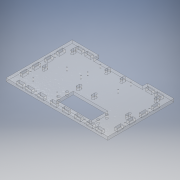
# Autodesk Inventor part: case_base
Saved by Autodesk Inventor 2019 (Build 230136000, 136)
## iProperties
Created: 2019-02-02
Part Number: case_base
Material: Acrylic, Clear
Document SubType Name: Modeling
Designer: suchanek
Density: 1.19 g/cm^3
Appearance: Transparent - Clear
Author: suchanek
Autodesk Inventor part; units mm, degrees
ref_plane "YZ Plane" through (0, 0, 0) normal (1, 0, 0) x (0, 1, 0)
ref_plane "XZ Plane" through (0, 0, 0) normal (0, 1, 0) x (-1, 0, 0)
ref_plane "XY Plane" through (0, 0, 0) normal (0, 0, 1) x (1, 0, 0)
sketch "Sketch1" plane through (0, 0, 0) normal (0, 1, 0) x (-1, 0, 0)
  line L0 (100, 65) -> (-100, 65)
  line L1 (-100, 65) -> (-100, -65)
  line L2 (-100, -65) -> (100, -65)
  line L3 (100, -65) -> (100, 65)
  line L4 (100, 65) -> (-100, -65) construction
  line L5 (-100, 65) -> (100, -65) construction
  line L6 (0, 0) -> (4.5236, 0)
  line L7 (0, 8.9) -> (0, -17.1)
  circle A0 centre (58.5, -13.1) radius 0.9
  circle A1 centre (30.6, -13.1) radius 0.9
  circle A2 centre (73.7, 37.7) radius 0.9
  circle A3 centre (25.5, 39) radius 0.9
  circle A4 centre (15, 6.45) radius 2.4
  line L8 (0, 0) -> (5.2635, 0)
  circle A5 centre (-15, 6.45) radius 2.4
  line L9 (48.5, 0) -> (48.5, 8.2763)
  line L10 (-48.5, 0) -> (-48.5, 8.2763)
  circle A6 centre (-82, 6.45) radius 2.4
  circle A7 centre (82, 6.45) radius 2.4
  line L11 (95.55, -41.85) -> (90.45, -41.85)
  line L12 (90.45, -41.85) -> (90.45, -30.15)
  line L13 (90.45, -30.15) -> (95.55, -30.15)
  line L14 (95.55, -30.15) -> (95.55, -41.85)
  line L15 (95.55, -17.85) -> (90.45, -17.85)
  line L16 (90.45, -17.85) -> (90.45, -6.15)
  line L17 (90.45, -6.15) -> (95.55, -6.15)
  line L18 (95.55, -6.15) -> (95.55, -17.85)
  line L19 (65.85, -55.45) -> (54.15, -55.45)
  line L20 (54.15, -55.45) -> (54.15, -60.55)
  line L21 (54.15, -60.55) -> (65.85, -60.55)
  line L22 (65.85, -60.55) -> (65.85, -55.45)
  line L23 (72.15, -60.55) -> (83.85, -60.55)
  line L24 (83.85, -60.55) -> (83.85, -55.45)
  line L25 (83.85, -55.45) -> (72.15, -55.45)
  line L26 (72.15, -55.45) -> (72.15, -60.55)
  line L27 (-95.55, -41.85) -> (-90.45, -41.85)
  line L28 (-90.45, -41.85) -> (-90.45, -30.15)
  line L29 (-90.45, -30.15) -> (-95.55, -30.15)
  line L30 (-95.55, -30.15) -> (-95.55, -41.85)
  line L31 (-95.55, -17.85) -> (-90.45, -17.85)
  line L32 (-90.45, -17.85) -> (-90.45, -6.15)
  line L33 (-90.45, -6.15) -> (-95.55, -6.15)
  line L34 (-95.55, -6.15) -> (-95.55, -17.85)
  line L35 (-65.85, -55.45) -> (-54.15, -55.45)
  line L36 (-54.15, -55.45) -> (-54.15, -60.55)
  line L37 (-54.15, -60.55) -> (-65.85, -60.55)
  line L38 (-65.85, -60.55) -> (-65.85, -55.45)
  line L39 (-72.15, -60.55) -> (-83.85, -60.55)
  line L40 (-83.85, -60.55) -> (-83.85, -55.45)
  line L41 (-83.85, -55.45) -> (-72.15, -55.45)
  line L42 (-72.15, -55.45) -> (-72.15, -60.55)
  line L43 (95.55, 41.85) -> (90.45, 41.85)
  line L44 (90.45, 41.85) -> (90.45, 30.15)
  line L45 (90.45, 30.15) -> (95.55, 30.15)
  line L46 (95.55, 30.15) -> (95.55, 41.85)
  line L47 (95.55, 17.85) -> (90.45, 17.85)
  line L48 (90.45, 17.85) -> (90.45, 6.15)
  line L49 (90.45, 6.15) -> (95.55, 6.15)
  line L50 (95.55, 6.15) -> (95.55, 17.85)
  line L51 (65.85, 55.45) -> (54.15, 55.45)
  line L52 (54.15, 55.45) -> (54.15, 60.55)
  line L53 (54.15, 60.55) -> (65.85, 60.55)
  line L54 (65.85, 60.55) -> (65.85, 55.45)
  line L55 (41.85, 55.45) -> (30.15, 55.45)
  line L56 (30.15, 55.45) -> (30.15, 60.55)
  line L57 (30.15, 60.55) -> (41.85, 60.55)
  line L58 (41.85, 60.55) -> (41.85, 55.45)
  line L59 (17.85, 55.45) -> (6.15, 55.45)
  line L60 (6.15, 55.45) -> (6.15, 60.55)
  line L61 (6.15, 60.55) -> (17.85, 60.55)
  line L62 (17.85, 60.55) -> (17.85, 55.45)
  line L63 (72.15, 60.55) -> (83.85, 60.55)
  line L64 (83.85, 60.55) -> (83.85, 55.45)
  line L65 (83.85, 55.45) -> (72.15, 55.45)
  line L66 (72.15, 55.45) -> (72.15, 60.55)
  line L67 (-90.45, 30.15) -> (-95.55, 30.15)
  line L68 (-95.55, 17.85) -> (-90.45, 17.85)
  line L69 (-90.45, 17.85) -> (-90.45, 6.15)
  line L70 (-90.45, 6.15) -> (-95.55, 6.15)
  line L71 (-95.55, 6.15) -> (-95.55, 17.85)
  line L72 (-95.55, 41.85) -> (-90.45, 41.85)
  line L73 (-95.55, 30.15) -> (-95.55, 41.85)
  line L74 (-90.45, 41.85) -> (-90.45, 30.15)
  line L75 (-83.85, 55.45) -> (-72.15, 55.45)
  line L76 (-83.85, 60.55) -> (-83.85, 55.45)
  line L77 (-72.15, 60.55) -> (-83.85, 60.55)
  line L78 (-72.15, 55.45) -> (-72.15, 60.55)
  line L79 (-65.85, 60.55) -> (-65.85, 55.45)
  line L80 (-54.15, 55.45) -> (-54.15, 60.55)
  line L81 (-54.15, 60.55) -> (-65.85, 60.55)
  line L82 (-65.85, 55.45) -> (-54.15, 55.45)
  line L83 (-6.15, 55.45) -> (-6.15, 60.55)
  line L84 (-17.85, 55.45) -> (-6.15, 55.45)
  line L85 (-6.15, 60.55) -> (-17.85, 60.55)
  line L86 (-17.85, 60.55) -> (-17.85, 55.45)
  line L87 (-30.15, 55.45) -> (-30.15, 60.55)
  line L88 (-41.85, 60.55) -> (-41.85, 55.45)
  line L89 (-30.15, 60.55) -> (-41.85, 60.55)
  line L90 (-41.85, 55.45) -> (-30.15, 55.45)
  line L91 (82, 3.95) -> (82, 8.95) construction
  line L92 (84.4, 3.95) -> (84.4, 8.95)
  line L93 (79.6, 8.95) -> (79.6, 3.95)
  arc A8 (79.6, 3.95) -> (84.4, 3.95) centre (82, 3.95) ccw
  arc A9 (84.4, 8.95) -> (79.6, 8.95) centre (82, 8.95) ccw
  line L94 (12.6, 3.95) -> (12.6, 8.95)
  line L95 (17.4, 8.95) -> (17.4, 3.95)
  arc A10 (12.6, 3.95) -> (17.4, 3.95) centre (15, 3.95) ccw
  arc A11 (17.4, 8.95) -> (12.6, 8.95) centre (15, 8.95) ccw
  line L96 (-84.4, 3.95) -> (-84.4, 8.95)
  line L97 (-79.6, 8.95) -> (-79.6, 3.95)
  arc A12 (-84.4, 3.95) -> (-79.6, 3.95) centre (-82, 3.95) ccw
  arc A13 (-79.6, 8.95) -> (-84.4, 8.95) centre (-82, 8.95) ccw
  arc A14 (-17.4, 3.95) -> (-12.6, 3.95) centre (-15, 3.95) ccw
  line L98 (-12.6, 3.95) -> (-12.6, 8.95)
  line L99 (-17.4, 8.95) -> (-17.4, 3.95)
  arc A15 (-12.6, 8.95) -> (-17.4, 8.95) centre (-15, 8.95) ccw
  line L100 (-56.5, 53.45) -> (11.5, 53.45)
  line L101 (11.5, 53.45) -> (11.5, 21.45)
  line L102 (11.5, 21.45) -> (-56.5, 21.45)
  line L103 (-56.5, 21.45) -> (-56.5, 53.45)
  circle A16 centre (-61.5, 28.45) radius 2.5
  circle A17 centre (-61.5, 45.45) radius 2.5
  line L104 (47.85, -65) -> (-47.85, -65)
  line L105 (-47.85, -65) -> (-47.85, -55.45)
  line L106 (-47.85, -55.45) -> (47.85, -55.45)
  line L107 (47.85, -55.45) -> (47.85, -65)
  line L108 (-22.5, 6.9) -> (-22.5, -4.1)
  circle A18 centre (16.5, 28.45) radius 2.5
  circle A19 centre (16.5, 45.45) radius 2.5
  circle A20 centre (30, -50.45) radius 0.9
  circle A21 centre (30, -25.45) radius 0.9
  circle A22 centre (-30, -25.45) radius 0.9
  circle A23 centre (-30, -50.45) radius 0.9
  circle A24 centre (93, -24) radius 1.125
  circle A25 centre (93, 24) radius 1.125
  circle A26 centre (-93, -24) radius 1.125
  circle A27 centre (-93, 24) radius 1.125
  circle A28 centre (48, 58) radius 1.125
  circle A29 centre (-48, 58) radius 1.125
  line L109 (65.3403, -21.55) -> (57.8403, -21.55)
  circle A30 centre (15, -49.55) radius 2.4
  circle A31 centre (-15, -49.55) radius 2.4
  circle A32 centre (-82, -49.55) radius 2.4
  circle A33 centre (82, -49.55) radius 2.4
  line L110 (82, -47.05) -> (82, -52.05) construction
  line L111 (84.4, -47.05) -> (84.4, -52.05)
  line L112 (79.6, -52.05) -> (79.6, -47.05)
  arc A34 (84.4, -47.05) -> (79.6, -47.05) centre (82, -47.05) ccw
  arc A35 (79.6, -52.05) -> (84.4, -52.05) centre (82, -52.05) ccw
  arc A36 (17.4, -47.05) -> (12.6, -47.05) centre (15, -47.05) ccw
  line L113 (12.6, -47.05) -> (12.6, -52.05)
  line L114 (17.4, -52.05) -> (17.4, -47.05)
  arc A37 (12.6, -52.05) -> (17.4, -52.05) centre (15, -52.05) ccw
  line L115 (-84.4, -47.05) -> (-84.4, -52.05)
  arc A38 (-84.4, -52.05) -> (-79.6, -52.05) centre (-82, -52.05) ccw
  line L116 (-79.6, -52.05) -> (-79.6, -47.05)
  arc A39 (-79.6, -47.05) -> (-84.4, -47.05) centre (-82, -47.05) ccw
  arc A40 (-12.6, -47.05) -> (-17.4, -47.05) centre (-15, -47.05) ccw
  line L117 (-17.4, -52.05) -> (-17.4, -47.05)
  line L118 (-12.6, -47.05) -> (-12.6, -52.05)
  arc A41 (-17.4, -52.05) -> (-12.6, -52.05) centre (-15, -52.05) ccw
  point P0 (0, 0)
  point P1 (0, 0)
  dimension "d0" = 130
  dimension "d1" = 200
  dimension "d7" = 1.8
  dimension "d8" = 5.1
  dimension "d9" = 27.9
  dimension "d10" = 1.3
  dimension "d11" = 50.8
  dimension "d12" = 15.2
  dimension "d14" = 26
  dimension "d23" = 4.8
  dimension "d31" = 5.1
  dimension "d32" = 4.45
  dimension "d34" = 6.15
  dimension "d35" = 11.7
  dimension "d36" = 12.3
  dimension "d37" = 11.7
  dimension "d43" = 11.7
  dimension "d44" = 6.3
  dimension "d45" = 11.7
  dimension "d50" = 2.5
  dimension "d54" = 10.5
  dimension "d55" = 32
  dimension "d56" = 68
  dimension "d58" = 5
  dimension "d62" = 17
  dimension "d63" = 5
  dimension "d64" = 12.3
  dimension "d65" = 11.7
  dimension "d66" = 5.1
  dimension "d67" = 12.3
  dimension "d68" = 11.7
  dimension "d69" = 12.3
  dimension "d70" = 11.7
  dimension "d71" = 12.3
  dimension "d72" = 11.7
  dimension "d73" = 4.45
  dimension "d74" = 6.3
  dimension "d75" = 6.3
  dimension "d77" = 15
  dimension "d78" = 67
  dimension "d79" = 5
  dimension "d80" = 25
  dimension "d81" = 60
  dimension "d82" = 2.25
  dimension "d83" = 6.15
  dimension "d84" = 2.55
  dimension "d85" = 2.25
  dimension "d86" = 2.25
  dimension "d87" = 2.55
  dimension "d88" = 6.15
  dimension "d89" = 7
  dimension "d90" = 56
  dimension "d91" = 15
  dimension "d92" = 2
  dimension "d93" = 22.5
  constraints: 242 end point, 104 symmetric about line, 42 centre point, 32 point on circle, 16 parallel, 14 point on line, 10 collinear, 10 horizontal, 8 equal radius, 8 vertical, 7 midpoint, 7 perpendicular, 5 tangent, 4 horizontal alignment, 3 vertical alignment, 28 other
  measures "d0" distance of L2.end L0.start
  measures "d1" distance of L1.end L2.end
  measures "d7" diameter of A1
  measures "d8" horizontal distance of A3.centre A1.centre
  measures "d9" distance of A1.centre A0.centre
  measures "d10" vertical distance of A2.centre A3.centre
  measures "d11" vertical distance of A0.centre A2.centre
  measures "d12" horizontal distance of A2.centre A0.centre
  measures "d14" distance from line of L0 A3.centre
  measures "d23" diameter of A4
  measures "d31" distance between parallel lines of L16 L18
  measures "d32" distance between parallel lines of L3 L18
  measures "d34" distance between parallel lines of L17 L8
  measures "d35" distance of L17.end L15.start
  measures "d36" distance between parallel lines of L15 L13
  measures "d37" distance of L13.end L11.start
  measures "d43" distance of L19.start L19.end
  measures "d44" distance between parallel lines of L22 L26
  measures "d45" distance of L24.end L25.end
  measures "d50" distance of A7.centre L91.end
  measures "d54" horizontal distance of A4.centre A3.centre
  measures "d55" distance of L100.end L101.end
  measures "d56" distance of L101.end L102.end
  measures "d58" distance from line of L103 A17.centre
  measures "d62" distance of A16.centre A17.centre
  measures "d63" diameter of A17
  measures "d64" distance between parallel lines of L58 L52
  measures "d65" distance of L56.end L58.start
  measures "d66" distance of L56.start L56.end
  measures "d67" distance between parallel lines of L62 L56
  measures "d68" distance of L61.start L62.start
  measures "d69" distance between parallel lines of L83 L60
  measures "d70" distance of L83.end L85.end
  measures "d71" distance between parallel lines of L87 L86
  measures "d72" distance of L87.end L89.end
  measures "d73" distance between parallel lines of L0 L61
  measures "d74" distance between parallel lines of L107 L20
  measures "d75" distance between parallel lines of L36 L105
  measures "d77" distance from line of L7 A4.centre
  measures "d78" distance of A6.centre A5.centre
  measures "d79" distance from line of L106 A20.centre
  measures "d80" distance of A20.centre A21.centre
  measures "d81" distance of A23.centre A20.centre
  measures "d82" diameter of A24
  measures "d83" distance from line of L13 A24.centre
  measures "d84" distance from line of L14 A24.centre
  measures "d85" diameter of A28
  measures "d86" diameter of A29
  measures "d87" distance from line of L53 A28.centre
  measures "d88" distance from line of L58 A28.centre
  measures "d89" distance from line of L102 A16.centre
  measures "d90" distance of A30.centre A4.centre
  measures "d91" distance from line of A5.centre L102
  measures "d92" distance between parallel lines of L84 L100
  measures "d93" distance between parallel lines of L7 L108
extrude "Extrusion3" add sketch "Sketch1" along normal blind 6 contours L3 L2 L107 L106 L105 L1 L0
body "Solid3"
